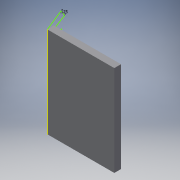
# Autodesk Inventor part: slide plate
Saved by Autodesk Inventor 2017 (Build 210142000, 142)
## iProperties
Created: 2016-12-09
Part Number: slide plate
Material: Generic
Document SubType Name: Modeling
Designer: Aditya
Density: 1 g/cm^3
Appearance: Default
Author: Aditya
Autodesk Inventor part; units mm, degrees
ref_plane "YZ Plane" through (0, 0, 0) normal (1, 0, 0) x (0, 1, 0)
ref_plane "XZ Plane" through (0, 0, 0) normal (0, 1, 0) x (-1, 0, 0)
ref_plane "XY Plane" through (0, 0, 0) normal (0, 0, 1) x (1, 0, 0)
sketch "Sketch1" plane through (0, 0, 0) normal (0, 0, 1) x (1, 0, 0)
  line L0 (0, 0) -> (31.75, 0)
  line L1 (31.75, 0) -> (31.75, 42.935)
  line L2 (31.75, 42.935) -> (0, 42.935)
  line L3 (0, 42.935) -> (0, 0)
  dimension "d0" = 31.75
  constraints: 8 end point, 3 perpendicular, 1 horizontal
  measures "d0" distance of L0.start L0.end
extrude "Extrusion1" add sketch "Sketch1" along normal blind 3.175
sketch "Sketch2" plane through (0, 0, 0) normal (-1, 0, 0) x (0, 0, 1)
  line L0 (-5.0008, 44.6006) -> (-1.6553, 42.6148)
  arc A0 (0, 40.2857) -> (-1.6553, 42.6148) centre (-3.4548, 39.5831) ccw
  line L1 (-5.0008, 44.6006) -> (-3.3281, 47.2993)
  line L2 (3.175, 0) -> (3.175, 42.935) projected
  line L3 (-3.3281, 47.2993) -> (3.175, 42.935)
  line L4 (0, 0) -> (0, 42.935) projected
  line L5 (0, 40.2857) -> (0, 42.935)
  line L6 (0, 42.935) -> (3.175, 42.935)
  dimension "d3" = 3.175
  constraints: 10 end point, 2 point on circle, 1 centre point, 1 collinear, 1 perpendicular, 1 tangent
  measures "d3" distance of L0.start L1.end
extrude "Extrusion2" add sketch "Sketch2" against normal blind 31.75
fillet "Fillet1" radius 6.35 1 edges at (15.875, 42.935, 3.175)
body "Solid1"
